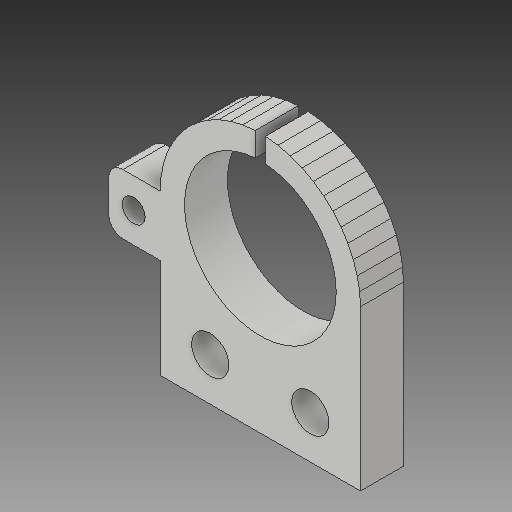
# Autodesk Inventor part: Left Bed Holder Upper
Saved by Autodesk Inventor 2017 (Build 210142000, 142)
## iProperties
Created: 2016-07-12
Part Number: Left Bed Holder Upper
Material: Generic
Document SubType Name: Modeling
Designer: joshmamo
Density: 1 g/cm^3
Appearance: Default
Author: joshmamo
Autodesk Inventor part; units mm, degrees
ref_plane "YZ Plane" through (0, 0, 0) normal (1, 0, 0) x (0, 1, 0)
ref_plane "XZ Plane" through (0, 0, 0) normal (0, 1, 0) x (-1, 0, 0)
ref_plane "XY Plane" through (0, 0, 0) normal (0, 0, 1) x (1, 0, 0)
sketch "Sketch1" plane through (0, 0, 0) normal (0, 0, 1) x (1, 0, 0)
  line L0 (-94.3346, 851.946) -> (-94.3346, 838.0325)
  line L1 (-94.3346, 838.0325) -> (-66.3346, 838.0325)
  line L2 (-66.3346, 838.0325) -> (-66.3346, 860.346)
  line L3 (-66.3346, 860.346) -> (-66.4468, 862.1155)
  line L4 (-66.4468, 862.1155) -> (-66.7819, 863.8566)
  line L5 (-66.7819, 863.8566) -> (-67.3343, 865.5414)
  line L6 (-67.3343, 865.5414) -> (-68.0952, 867.1429)
  line L7 (-68.0952, 867.1429) -> (-69.0524, 868.6354)
  line L8 (-69.0524, 868.6354) -> (-70.1906, 869.9949)
  line L9 (-70.1906, 869.9949) -> (-71.4915, 871.1996)
  line L10 (-71.4915, 871.1996) -> (-72.9342, 872.2303)
  line L11 (-72.9342, 872.2303) -> (-74.4956, 873.0703)
  line L12 (-74.4956, 873.0703) -> (-76.1507, 873.7063)
  line L13 (-76.1507, 873.7063) -> (-77.8729, 874.1279)
  line L14 (-77.8729, 874.1279) -> (-79.6346, 874.3285)
  line L15 (-79.6346, 874.3285) -> (-79.6346, 870.8227)
  line L16 (-79.6346, 870.8227) -> (-77.9981, 870.5828)
  line L17 (-77.9981, 870.5828) -> (-76.4195, 870.0889)
  line L18 (-76.4195, 870.0889) -> (-74.9382, 869.3532)
  line L19 (-74.9382, 869.3532) -> (-73.5907, 868.394)
  line L20 (-73.5907, 868.394) -> (-72.4106, 867.2352)
  line L21 (-72.4106, 867.2352) -> (-71.427, 865.9054)
  line L22 (-71.427, 865.9054) -> (-70.6646, 864.4376)
  line L23 (-70.6646, 864.4376) -> (-70.142, 862.8683)
  line L24 (-70.142, 862.8683) -> (-69.8724, 861.2365)
  line L25 (-69.8724, 861.2365) -> (-69.8623, 859.5825)
  line L26 (-69.8623, 859.5825) -> (-70.1122, 857.9475)
  line L27 (-70.1122, 857.9475) -> (-70.6156, 856.372)
  line L28 (-70.6156, 856.372) -> (-71.3603, 854.8951)
  line L29 (-71.3603, 854.8951) -> (-72.3276, 853.5535)
  line L30 (-72.3276, 853.5535) -> (-73.4936, 852.3804)
  line L31 (-73.4936, 852.3804) -> (-74.8293, 851.405)
  line L32 (-74.8293, 851.405) -> (-76.3017, 850.6514)
  line L33 (-76.3017, 850.6514) -> (-77.8741, 850.1384)
  line L34 (-77.8741, 850.1384) -> (-79.5076, 849.8787)
  line L35 (-79.5076, 849.8787) -> (-81.1615, 849.8787)
  line L36 (-81.1615, 849.8787) -> (-82.795, 850.1384)
  line L37 (-82.795, 850.1384) -> (-84.3674, 850.6514)
  line L38 (-84.3674, 850.6514) -> (-85.8398, 851.405)
  line L39 (-85.8398, 851.405) -> (-87.1755, 852.3804)
  line L40 (-87.1755, 852.3804) -> (-88.3415, 853.5535)
  line L41 (-88.3415, 853.5535) -> (-89.3088, 854.8951)
  line L42 (-89.3088, 854.8951) -> (-90.0535, 856.372)
  line L43 (-90.0535, 856.372) -> (-90.5569, 857.9475)
  line L44 (-90.5569, 857.9475) -> (-90.8068, 859.5825)
  line L45 (-90.8068, 859.5825) -> (-90.7967, 861.2365)
  line L46 (-90.7967, 861.2365) -> (-90.5271, 862.8683)
  line L47 (-90.5271, 862.8683) -> (-90.0046, 864.4376)
  line L48 (-90.0046, 864.4376) -> (-89.2421, 865.9054)
  line L49 (-89.2421, 865.9054) -> (-88.2586, 867.2352)
  line L50 (-88.2586, 867.2352) -> (-87.0784, 868.394)
  line L51 (-87.0784, 868.394) -> (-85.731, 869.3532)
  line L52 (-85.731, 869.3532) -> (-84.2496, 870.0889)
  line L53 (-84.2496, 870.0889) -> (-82.6711, 870.5828)
  line L54 (-82.6711, 870.5828) -> (-81.0346, 870.8227)
  line L55 (-81.0346, 870.8227) -> (-81.0346, 874.3285)
  line L56 (-81.0346, 874.3285) -> (-82.7962, 874.1279)
  line L57 (-82.7962, 874.1279) -> (-84.5184, 873.7063)
  line L58 (-84.5184, 873.7063) -> (-86.1735, 873.0703)
  line L59 (-86.1735, 873.0703) -> (-87.7349, 872.2303)
  line L60 (-87.7349, 872.2303) -> (-89.1776, 871.1996)
  line L61 (-89.1776, 871.1996) -> (-90.4785, 869.9949)
  line L62 (-90.4785, 869.9949) -> (-91.6167, 868.6354)
  line L63 (-91.6167, 868.6354) -> (-92.5739, 867.1429)
  line L64 (-92.5739, 867.1429) -> (-93.3349, 865.5414)
  line L65 (-93.3349, 865.5414) -> (-93.8873, 863.8566)
  line L66 (-93.8873, 863.8566) -> (-94.2223, 862.1155)
  line L67 (-94.2223, 862.1155) -> (-94.3346, 860.346)
  line L68 (-94.3346, 860.346) -> (-99.5495, 860.346)
  arc A0 (-99.5495, 860.346) -> (-101.5495, 858.346) centre (-99.5495, 858.346) ccw
  line L69 (-101.5495, 858.346) -> (-101.5495, 853.946)
  arc A1 (-101.5495, 853.946) -> (-99.5495, 851.946) centre (-99.5495, 853.946) ccw
  line L70 (-99.5495, 851.946) -> (-94.3346, 851.946)
  circle A2 centre (-98.0495, 856.146) radius 1.6
  circle A3 centre (-87.3346, 844.0325) radius 2.6
  circle A4 centre (-73.3346, 844.0325) radius 2.6
  point P0 (0, 0)
  constraints: 142 end point, 5 centre point, 4 point on circle
extrude "Extrusion1" add sketch "Sketch1" along normal blind 6
sketch "Sketch3" plane through (0, 0, 0) normal (0, 0, -1) x (-1, 0, 0)
  line L0 (69.8724, 861.2365) -> (69.8623, 859.5825) projected
  line L1 (69.8674, 860.4095) -> (90.8017, 860.4095)
  line L2 (90.8068, 859.5825) -> (90.7967, 861.2365) projected
  point P0 (0, 0)
  point P1 (80.3346, 860.4095)
  constraints: 3 midpoint, 2 end point
hole "Hole1" at (-80.3346, 860.4095, 0) direction (0, 0, 1) diameter 21.2 depth 8 tip angle 118
body "Solid1"
